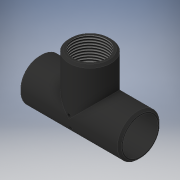
# Autodesk Inventor part: penyambung
Saved by Autodesk Inventor 2019.5 (Build 235369000, 369)
## iProperties
Created: 2022-10-10
Part Number: penyambung
Material: Rubber, Silicone
Document SubType Name: Modeling
Designer: ASUS
Density: 1.25 g/cm^3
Appearance: Rubber - Black
Author: ASUS
Autodesk Inventor part; units mm, degrees
ref_plane "YZ Plane" through (0, 0, 0) normal (1, 0, 0) x (0, 1, 0)
ref_plane "XZ Plane" through (0, 0, 0) normal (0, 1, 0) x (-1, 0, 0)
ref_plane "XY Plane" through (0, 0, 0) normal (0, 0, 1) x (1, 0, 0)
sketch "Sketch2" plane through (0, 0, 0) normal (0, 0, 1) x (1, 0, 0)
  line L0 (60, 0) -> (60, 60)
  line L1 (0, 0) -> (0, -25)
  line L2 (0, -25) -> (120, -25)
  line L3 (120, -25) -> (120, 0)
  line L4 (60, 60) -> (85, 60)
  line L5 (85, 60) -> (85, 0)
  line L6 (60, 0) -> (85, 0)
  line L7 (0, 0) -> (120, 0)
  dimension "d4" = 120
  dimension "d5" = 60
  dimension "d6" = 25
  dimension "d7" = 25
  constraints: 16 end point, 3 perpendicular, 2 vertical, 1 horizontal
  measures "d4" distance of L1.start L3.end
  measures "d5" distance of L0.start L0.end
  measures "d6" distance of L1.start L1.end
  measures "d7" distance of L0.end L4.end
revolve "Revolution1" add sketch "Sketch2" angle 360 about axis through (0, 0, 0) along (1, 0, 0) contours L6 L7 L3 L2 L1
revolve "Revolution2" add sketch "Sketch2" angle 360 about axis through (60, 0, 0) along (0, 1, 0) contours L0 L4 L5 L6
sketch "Sketch3" plane through (60, 60, 0) normal (0, 1, 0) x (1, 0, 0)
  point P0 (-60, 0)
  point P1 (0.0519, -0.0386)
hole "Hole1" at (60.0519, 60, 0.0386) direction (0, -1, 0) diameter 40 depth 35
shell "Shell1" thickness 4 removed faces 2 at (120, -4.976, 4.8639) at (0, 0.7623, 6.2783)
chamfer "Chamfer1" distance 2.5 angle 45 3 edges at (0, 25, 0) (120, 25, 0) (35, 60, 0)
thread "Thread1" size "M40x3" class "6H" standard "ANSI Metric M Profile" full length
sketch "Sketch4" plane through (0, 0, 0) normal (0, 0, 1) x (1, 0, 0)
  line L0 (0, 0) -> (130.4207, 0)
  circle A0 centre (60, -10.0213) radius 1.5
  circle A1 centre (60, 3.7799) radius 1.5
  dimension "d23" = 3
  dimension "d36" = 3
  constraints: 2 centre point, 2 end point, 1 horizontal
  measures "d23" diameter of A0
  measures "d36" diameter of A1
extrude "Extrusion2" add sketch "Sketch4" along normal blind 54.5 contours A0
extrude "Extrusion3" add sketch "Sketch4" along normal blind 54.5 contours A1
sketch "Sketch6" plane through (60, -10.0213, 54.5) normal (0, 0, 1) x (1, 0, 0)
  point P0 (-60, 10.0213)
  point P1 (-0.0413, -0.0123)
hole "Hole3" at (59.9587, -10.0336, 54.5) direction (0, 0, -1) diameter 4 depth 55.5
sketch "Sketch7" plane through (60, 3.7799, 54.5) normal (0, 0, 1) x (1, 0, 0)
  point P0 (-60, -3.7799)
  point P1 (0.0079, -0.0109)
hole "Hole4" at (60.0079, 3.769, 54.5) direction (0, 0, -1) diameter 4 depth 55.5
body "Solid1"
